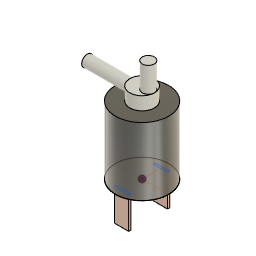
_ 12V valve v2 (Autodesk Fusion 360 design; units mm, degrees)
Autodesk Fusion 360 part; units mm, degrees
sketch "Sketch1" plane through (0, 0, 0) normal (0, 0, 1) x (1, 0, 0)
  circle A0 centre (0, 0) radius 11.8
  line L0 (0, 0) -> (11.8, 0) construction
  line L1 (0, 11.8) -> (0, 0) construction
  line L2 (-3.15, 8.1) -> (-3.15, 9.1)
  line L3 (3.15, 8.1) -> (-3.15, 8.1)
  line L4 (-3.15, 9.1) -> (3.15, 9.1)
  line L5 (3.15, 9.1) -> (3.15, 8.1)
  line L6 (-3.15, -9.1) -> (3.15, -9.1)
  line L7 (3.15, -9.1) -> (3.15, -8.1)
  line L8 (3.15, -8.1) -> (-3.15, -8.1)
  line L9 (-3.15, -8.1) -> (-3.15, -9.1)
  dimension "d1" = 23.6
  dimension "d19" = 1
  dimension "d20" = 6.3
  dimension "d21" = 9.1
  constraint coincident A0.centre L0.start
  constraint coincident A0 L0.end
  constraint coincident A0 L1.start
  constraint perpendicular L0 L1
  constraint symmetric L0 L2.end L6.start
  constraint symmetric L0 L2.start L8.end
  measures "d1" diameter of A0
  measures "d19" distance of L3 L4
  measures "d20" distance of L2 L5
  measures "d21" distance of L0 L4
extrude "Extrude1" add sketch "Sketch1" along normal blind 30 contours A0 | L2 L3 L4 L5 | L6 L7 L8 L9 makes body 1
extrude "Extrude2" add sketch "Sketch1" against normal blind 14 separate body contours L2 L3 L4 L5 | L6 L7 L8 L9 makes body 2 at (1.05, -8.1, -4.6667) makes body 3 at (-1.05, 9.1, -4.6667)
sketch "Sketch2" plane through (0, 0, 30) normal (0, 0, 1) x (-1, 0, 0)
  circle A0 centre (0, 0) radius 11.8
  circle A1 centre (0, 0) radius 5.45
  dimension "d10" = 10.9
  constraint concentric A0 A1
  measures "d10" diameter of A1
extrude "Extrude3" add sketch "Sketch2" along normal blind 5.8 separate body contours A1 makes body 4
sketch "Sketch3" plane through (0, 0, 35.8) normal (0, 0, 1) x (-1, 0, 0)
  circle A0 centre (0, 0) radius 5.45
  circle A1 centre (-2.75, 0) radius 2.7
  line L0 (0, 0) -> (-11.8, 0)
  dimension "d13" = 5.4
  constraint coincident A1.centre L0
  constraint tangent A0 A1
  measures "d13" diameter of A1
extrude "Extrude4" add sketch "Sketch3" along normal blind 11.1 contours A1 L0 | A1 L0 bodies 4
sketch "Sketch4" plane through (0, 0, 0) normal (1, 0, 0) x (0, 1, 0)
  circle A0 centre (0, 33.3) radius 2.5
  line L0 (5.45, 35.8) -> (-5.45, 35.8)
  dimension "d16" = 5
  constraint tangent A0 L0
  measures "d16" diameter of A0
extrude "Extrude5" add sketch "Sketch4" against normal blind 24.3 bodies 4
